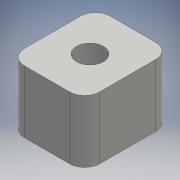
# Autodesk Inventor part: платик под двигатель
Saved by Autodesk Inventor 2016 (Build 200138000, 138)
## iProperties
Created: 2021-05-08
Part Number: платик под двигатель
Material: Типовые
Document SubType Name: Modeling
Designer: Лол
Density: 1 g/cm^3
Appearance: По умолчанию
Author: Лол
Autodesk Inventor part; units mm, degrees
ref_plane "YZ Plane" through (0, 0, 0) normal (1, 0, 0) x (0, 1, 0)
ref_plane "XZ Plane" through (0, 0, 0) normal (0, 1, 0) x (-1, 0, 0)
ref_plane "XY Plane" through (0, 0, 0) normal (0, 0, 1) x (1, 0, 0)
sketch "Эскиз1" plane through (0, 0, 0) normal (0, 0, 1) x (1, 0, 0)
  line L0 (17.5, -20) -> (-17.5, -20)
  line L1 (-17.5, -20) -> (-17.5, 20)
  line L2 (-17.5, 20) -> (17.5, 20)
  line L3 (17.5, 20) -> (17.5, -20)
  line L4 (17.5, -20) -> (-17.5, 20) construction
  line L5 (-17.5, -20) -> (17.5, 20) construction
  circle A0 centre (0, 0) radius 6.25
  dimension "d0" = 40
  dimension "d1" = 12.5
  dimension "d11" = 35
  constraints: 12 end point, 2 midpoint, 2 parallel, 1 centre point, 1 coincident, 1 horizontal, 1 perpendicular
  measures "d0" distance of L2.end L0.start
  measures "d1" diameter of A0
  measures "d11" distance between parallel lines of L1 L3
extrude "Выдавливание1" add sketch "Эскиз1" along normal blind 29
fillet "Сопряжение1" radius 7 4 edges at (-17.5, -20, 14.5) (-17.5, 20, 14.5) (17.5, 20, 14.5) (17.5, -20, 14.5)
sketch "Эскиз2" plane through (0, 0, 0) normal (0, 0, -1) x (-1, 0, 0)
  line L0 (-10.5, -20) -> (10.5, -20) projected
  line L1 (10.5, 20) -> (-10.5, 20) projected
  line L2 (-17.5, 13) -> (-17.5, -13) projected
  arc A0 (-17.5, -13) -> (-10.5, -20) centre (-10.5, -13) ccw projected
  arc A1 (10.5, -20) -> (17.5, -13) centre (10.5, -13) ccw projected
  arc A2 (17.5, 13) -> (10.5, 20) centre (10.5, 13) ccw projected
  arc A3 (-10.5, 20) -> (-17.5, 13) centre (-10.5, 13) ccw projected
  line L3 (17.5, -13) -> (17.5, 13) projected
  line L4 (-12.5, 15) -> (12.5, 15)
  line L5 (12.5, 15) -> (12.5, -15)
  line L6 (12.5, -15) -> (-12.5, -15)
  line L7 (-12.5, -15) -> (-12.5, 15)
  line L8 (-12.5, 15) -> (12.5, -15) construction
  line L9 (12.5, 15) -> (-12.5, -15) construction
  point P0 (0, 0)
  dimension "d12" = 5
  dimension "d13" = 5
  constraints: 12 end point, 2 midpoint, 2 parallel, 1 horizontal, 1 perpendicular
  measures "d12" distance between parallel lines of L0 L6
  measures "d13" distance between parallel lines of L3 L5
extrude "Выдавливание2" cut sketch "Эскиз2" against normal blind 5 contours L4 L5 L6 L7
fillet "Сопряжение3" radius 2 4 edges at (12.5, -15, 2.5) (-12.5, -15, 2.5) (-12.5, 15, 2.5) (12.5, 15, 2.5)
